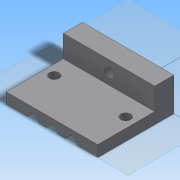
# Autodesk Inventor part: keyhole holder
Saved by Autodesk Inventor 2014 SP2 (Build 180246200, 246)
## iProperties
Created: 2014-06-06
Part Number: keyhole holder
Material: Generic
Document SubType Name: Modeling
Designer: dliu
Density: 1 g/cm^3
Appearance: Default
Author: dliu
Autodesk Inventor part; units mm, degrees
ref_plane "YZ Plane" through (0, 0, 0) normal (1, 0, 0) x (0, 1, 0)
ref_plane "XZ Plane" through (0, 0, 0) normal (0, 1, 0) x (-1, 0, 0)
ref_plane "XY Plane" through (0, 0, 0) normal (0, 0, 1) x (1, 0, 0)
sketch "Sketch1" plane through (0, 0, 0) normal (0, 0, 1) x (1, 0, 0)
  circle A0 centre (-6.35, 0) radius 2.2543
  circle A1 centre (0, 0) radius 2.2543
  circle A2 centre (6.35, 0) radius 2.2543
  line L0 (-15.24, 3.81) -> (15.24, 3.81)
  line L1 (15.24, 3.81) -> (15.24, 0)
  line L2 (15.24, 0) -> (-15.24, 0)
  line L3 (-15.24, 0) -> (-15.24, 3.81)
  dimension "d0" = 4.5085
  dimension "d3" = 6.35
  dimension "d4" = 6.35
  dimension "d5" = 3.81
  dimension "d6" = 30.48
  constraints: 8 end point, 3 centre point, 3 horizontal alignment, 2 equal radius, 2 parallel, 1 coincident, 1 horizontal, 1 midpoint, 1 perpendicular
  measures "d0" diameter of A0
  measures "d3" distance of A1.centre A0.centre
  measures "d4" distance of A2.centre A1.centre
  measures "d5" distance of L2.end L0.start
  measures "d6" distance of L0.start L0.end
extrude "Extrusion1" add sketch "Sketch1" along normal blind 25.4 contours L2 A0 | A0 L2 L3 L0 L1 A2 A1 | A1 L2 | A2 L2 picked at (-7.1014, 0.9966) picked at (0.5625, 0.4983) picked at (6.8906, 0.6781)
extrude "Extrusion2" cut sketch "Sketch1" along normal blind 20.574 contours L2 A0 | A0 L2 | L2 A1 | A1 L2 | L2 A2 | A2 L2
sketch "Sketch2" plane through (0, 0, 25.4) normal (0, 0, 1) x (1, 0, 0)
  circle A0 centre (0, 0) radius 2.2543 projected
  circle A1 centre (6.35, 0) radius 2.2543 projected
  circle A2 centre (-6.35, 0) radius 2.2543 projected
  circle A3 centre (-6.35, 0) radius 2.032
  circle A4 centre (0, 0) radius 2.032
  circle A5 centre (6.35, 0) radius 2.032
  dimension "d11" = 4.064
  constraints: 3 centre point, 3 coincident, 2 equal radius
  measures "d11" diameter of A3
extrude "Extrusion3" cut sketch "Sketch2" against normal blind 4.826 contours A3 | A4 | A5
sketch "Sketch3" plane through (0, 0, 0) normal (0, 1, 0) x (-1, 0, 0)
  line L0 (15.24, 0) -> (-15.24, 0) construction
  line L1 (15.24, 0) -> (15.24, 25.4) construction
  line L2 (-15.24, 25.4) -> (15.24, 25.4) construction
  line L3 (-15.24, 0) -> (-15.24, 25.4) construction
  line L4 (-15.24, 12.7) -> (15.24, 12.7) construction
  line L5 (-8.6043, 20.574) -> (-8.6043, 0) construction
  line L6 (-11.9221, 12.7) -> (-8.6043, 12.7)
  line L7 (-11.9221, 12.7) -> (-15.24, 12.7)
  constraints: 6 end point, 3 point on line, 2 collinear, 2 midpoint
hole "Hole1" at (11.9221, 0, 12.7) direction (0, 1, 0) diameter 3.2766 end through all clearance for "Oval Head Machine Screw" size "#4" standard "Ansi Unified Screw Threads"
mirror "Mirror1" about plane through (0, 0, 0) normal (1, 0, 0) of "Hole1"
sketch "Sketch7" plane through (0, 0, 0) normal (0, 0, 1) x (1, 0, 0)
  line L0 (-15.24, 3.81) -> (15.24, 3.81) projected
  line L1 (15.24, 3.81) -> (-15.24, 3.81)
  line L2 (-15.24, 3.81) -> (-15.24, 11.176)
  line L3 (-15.24, 11.176) -> (15.24, 11.176)
  line L4 (15.24, 11.176) -> (15.24, 3.81)
  line L5 (-15.24, 7.493) -> (15.24, 7.493)
  point P0 (0, 7.493)
  point P1 (0, 0)
  point P2 (0, 7.493)
  dimension "d36" = 3.683
  constraints: 10 end point, 3 midpoint, 2 parallel, 1 coincident, 1 horizontal, 1 perpendicular, 1 vertical alignment
  measures "d36" distance from line of L0 point (0, 7.493)
extrude "Extrusion5" add sketch "Sketch7" along normal blind 6.35
hole "Hole2" at (0, 7.493, 0) direction (0, 0, 1) diameter 3.2766 end through all clearance for "Oval Head Machine Screw" size "#4" standard "Ansi Unified Screw Threads"
body "Solid1"
